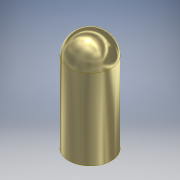
# Autodesk Inventor part: Plunger
Saved by Autodesk Inventor 2018 (Build 220112000, 112)
## iProperties
Created: 2018-11-03
Part Number: Plunger
Material: Nickel-Copper Alloy 400
Document SubType Name: Modeling
Designer: Bradley
Density: 8.83 g/cm^3
Appearance: Gold - Metal
Author: Bradley
Autodesk Inventor part; units mm, degrees
ref_plane "YZ Plane" through (0, 0, 0) normal (1, 0, 0) x (0, 1, 0)
ref_plane "XZ Plane" through (0, 0, 0) normal (0, 1, 0) x (-1, 0, 0)
ref_plane "XY Plane" through (0, 0, 0) normal (0, 0, 1) x (1, 0, 0)
sketch "Sketch1" plane through (0, 0, 0) normal (0, 1, 0) x (-1, 0, 0)
  line L0 (0, -1.27) -> (0, 1.27)
  arc A0 (0, 1.27) -> (-0.5334, 0.7366) centre (0, 0.7366) ccw
  line L1 (-0.5334, 0.7366) -> (-0.5334, -1.27)
  line L2 (-0.5334, -1.27) -> (0, -1.27)
  point P0 (0, 0)
  point P1 (0, 0)
  dimension "d0" = 1.0668
  dimension "d1" = 2.54
  constraints: 6 end point, 2 point on circle, 1 centre point, 1 coincident, 1 midpoint, 1 parallel, 1 perpendicular, 1 point on line, 1 tangent, 1 vertical
  measures "d0" diameter of L1 L0
  measures "d1" distance of L0.start L0.end
revolve "Revolution1" add sketch "Sketch1" angle 360 about axis through (0, 0, -1.27) along (0, 0, 1)
body "Solid1"
